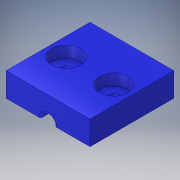
# Autodesk Inventor part: TopOfSquareSupport
Saved by Autodesk Inventor 2017 SP1 (Build 210196100, 196)
## iProperties
Created: 2015-12-11
Part Number: TopOfSquareSupport
Material: PC/ABS Plastic
Document SubType Name: Modeling
Designer: steele
Density: 0.357273 g/cm^3
Appearance: Blue - Wall Paint - Glossy
Author: steele
Autodesk Inventor part; units mm, degrees
ref_plane "YZ Plane" through (0, 0, 0) normal (1, 0, 0) x (0, 1, 0)
ref_plane "XZ Plane" through (0, 0, 0) normal (0, 1, 0) x (-1, 0, 0)
ref_plane "XY Plane" through (0, 0, 0) normal (0, 0, 1) x (1, 0, 0)
sketch "Sketch5" plane through (0, 0, 0) normal (0, 1, 0) x (-1, 0, 0)
  line L0 (-22.225, 22.225) -> (-22.225, -22.225)
  line L1 (-22.225, -22.225) -> (22.225, -22.225)
  line L2 (22.225, -22.225) -> (22.225, 22.225)
  line L3 (22.225, 22.225) -> (-22.225, 22.225)
  line L4 (-22.225, 22.225) -> (22.225, -22.225) construction
  line L5 (-22.225, -22.225) -> (22.225, 22.225) construction
  point P0 (0, 0)
  dimension "d23" = 44.45
  constraints: 12 end point, 2 midpoint, 2 parallel, 2 perpendicular, 1 vertical
  measures "d23" distance of L0.start L0.end
extrude "Extrusion3" add sketch "Sketch5" along normal blind 12.7
sketch "Sketch6" plane through (-22.225, 0, 22.225) normal (0, 0, 1) x (1, 0, 0)
  point P0 (22.225, 0)
  point P1 (22.225, 0)
  constraints: 1 coincident
hole "Hole2" at (0, 0, 22.225) direction (0, 0, -1) diameter 6.35 end through all
sketch "Sketch7" plane through (0, 12.7, 0) normal (0, 1, 0) x (1, 0, 0)
  line L0 (-22.225, 22.225) -> (-22.225, -22.225) projected
  line L1 (22.225, -22.225) -> (22.225, 22.225) projected
  line L2 (-22.225, -22.225) -> (22.225, -22.225) projected
  point P0 (0, 0)
  point P1 (-12.7, 0)
  point P2 (12.7, 0)
  dimension "d33" = 9.525
  dimension "d34" = 9.525
  dimension "d53" = 22.225
  dimension "d54" = 22.225
  measures "d33" distance from line of point (-12.7, 0) L0
  measures "d34" distance from line of point (12.7, 0) L1
  measures "d53" distance from line of L2 point (-12.7, 0)
  measures "d54" distance from line of L2 point (12.7, 0)
hole "Hole3" at (-12.7, 12.7, 0) at (12.7, 12.7, 0) direction (0, -1, 0) diameter 15.24 depth 6.096
sketch "Sketch8" plane through (0, 12.7, 0) normal (0, 1, 0) x (1, 0, 0)
  line L0 (-22.225, 22.225) -> (-22.225, -22.225) projected
  line L1 (22.225, -22.225) -> (22.225, 22.225) projected
  line L2 (-22.225, -22.225) -> (22.225, -22.225) projected
  point P0 (0, 0)
  point P1 (-12.7, 0)
  point P2 (12.7, 0)
  dimension "d42" = 9.525
  dimension "d43" = 9.525
  dimension "d51" = 22.225
  dimension "d52" = 22.225
  measures "d42" distance from line of point (-12.7, 0) L0
  measures "d43" distance from line of L1 point (12.7, 0)
  measures "d51" distance from line of L2 point (-12.7, 0)
  measures "d52" distance from line of L2 point (12.7, 0)
hole "Hole4" at (-12.7, 12.7, 0) at (12.7, 12.7, 0) direction (0, -1, 0) diameter 5.6134 end through all clearance for "Flat Head Machine Screw (82)" size "#10" standard "Ansi Unified Screw Threads"
sketch "Sketch9" plane through (0, 0, 0) normal (0, -1, 0) x (1, 0, 0)
  line L0 (-12.7, -12.7) -> (12.7, -12.7) construction
  line L1 (12.7, -12.7) -> (12.7, 12.7) construction
  line L2 (12.7, 12.7) -> (-12.7, 12.7) construction
  line L3 (-12.7, 12.7) -> (-12.7, -12.7) construction
  line L4 (-12.7, -12.7) -> (12.7, 12.7) construction
  line L5 (12.7, -12.7) -> (-12.7, 12.7) construction
  line L6 (-3.175, -22.225) -> (-22.225, -22.225) construction
  line L7 (-22.225, -22.225) -> (-22.225, 22.225) construction
  circle A0 centre (-12.7, -12.7) radius 2.7305
  circle A1 centre (12.7, -12.7) radius 2.7305
  circle A2 centre (12.7, 12.7) radius 2.7305
  circle A3 centre (-12.7, 12.7) radius 2.7305
  point P0 (0, 0)
  dimension "d55" = 9.525
  dimension "d56" = 9.525
  dimension "d57" = 5.461
  constraints: 12 end point, 4 centre point, 4 coincident, 3 equal radius, 2 midpoint, 2 parallel, 1 horizontal, 1 perpendicular
  measures "d55" distance between parallel lines of L6 L0
  measures "d56" distance between parallel lines of L7 L3
  measures "d57" diameter of A0
extrude "Extrusion4" add sketch "Sketch9" along normal blind 5.08
fillet "Fillet1" radius 1.5875 4 edges at (-15.4305, -5.08, 12.7) (9.9695, -5.08, 12.7) (9.9695, -5.08, -12.7) (-15.4305, -5.08, -12.7)
fillet "Fillet2" radius 1.5875 4 edges at (3.175, 0, 0) (-3.175, 0, 0) (0, 3.175, 22.225) (0, 3.175, -22.225)
equation "\"d23\" = basewidth"
equation "\"d24\" = heightOfTopSection"
equation "\"d26\" = topHoleDiam"
equation "\"d33\" = edgeToBoltHole"
equation "\"d34\" = edgeToBoltHole"
equation "\"d53\" = 0.5 * basewidth"
equation "\"d54\" = 0.5 * basewidth"
equation "\"d35\" = washerDiam"
equation "\"d40\" = depthForSocketHead"
equation "\"d42\" = edgeToBoltHole"
equation "\"d43\" = edgeToBoltHole"
equation "\"d51\" = 0.5 * basewidth"
equation "\"d52\" = 0.5 * basewidth"
equation "\"d55\" = edgeToBoltHole"
equation "\"d56\" = edgeToBoltHole"
equation "\"d57\" = supportHoleDiam"
equation "\"d58\" = supportHoleLength"
equation "\"bottomHoleDiam\" = 6.35"
equation "\"basewidth\" = 44.45"
equation "\"deltaBottomToTop\" = 25.4"
equation "\"d0\" = basewidth"
equation "\"d1\" = heightOfBottomHole"
equation "\"d2\" = 0"
equation "\"d3\" = bottomHoleDiam"
equation "\"d5\" = 0"
equation "\"topHoleDiam\" = bottomHoleDiam"
equation "\"height\" = deltaBottomToTop + heightOfBottomHole + heightOfTopHole"
equation "\"heightOfTopSection\" = 12.7"
equation "\"edgeToBoltHole\" = -0.25 * bottomHoleDiam + 0.25 * basewidth"
equation "\"washerDiam\" = 15.24"
equation "\"depthForSocketHead\" = 6.096"
equation "\"heightOfTopSupport\" = 12.7"
equation "\"baseLength\" = 44.45"
equation "\"supportHoleDiam\" = 5.461"
equation "\"supportHoleLength\" = 5.08"
equation "\"heightOfBottomHole\" = 9.525"
equation "\"heightOfTopHole\" = 9.525"
body "Solid2"
